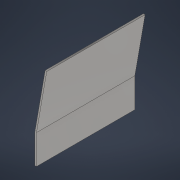
# Autodesk Inventor part: SteelBack
Saved by Autodesk Inventor 2021 (Build 250183000, 183)
## iProperties
Created: 2021-01-30
Part Number: SteelBack
Material: Generic
Document SubType Name: Modeling
Designer: argon
Density: 1 g/cm^3
Appearance: Steel - Polished
Author: argon
Autodesk Inventor part; units mm, degrees
ref_plane "YZ Plane" through (0, 0, 0) normal (1, 0, 0) x (0, 1, 0)
ref_plane "XZ Plane" through (0, 0, 0) normal (0, 1, 0) x (-1, 0, 0)
ref_plane "XY Plane" through (0, 0, 0) normal (0, 0, 1) x (1, 0, 0)
sketch "Sketch1" plane through (0, 0, 0) normal (0, 0, 1) x (1, 0, 0)
  line L0 (0, 0) -> (0, 118.2502)
  line L1 (0.3038, 121.7232) -> (41.6756, 356.3539)
  arc A0 (0.3038, 121.7232) -> (0, 118.2502) centre (20, 118.2502) ccw
  line L2 (47.9291, 355.2512) -> (6.35, 119.4444)
  line L3 (6.35, 119.4444) -> (6.35, 0)
  line L4 (41.6756, 356.3539) -> (47.9291, 355.2512)
  line L5 (0, 0) -> (6.35, 0)
  point P0 (0, 120)
  dimension "d0" = 170
  dimension "d1" = 120
  dimension "d2" = 240
  dimension "d3" = 20
  dimension "d4" = 6.35
  constraints: 12 end point, 2 perpendicular, 2 point on circle, 2 point on line, 2 tangent, 1 centre point, 1 horizontal, 1 other
  measures "d0" angle of L0 L1
  measures "d1" distance of L0.start point (0, 120)
  measures "d2" distance of point (0, 120) L1.end
  measures "d3" radius of A0
  measures "d4" distance between parallel lines of L2 L1
extrude "Extrusion1" add sketch "Sketch1" along normal blind 400
body "Solid1"
